Autodesk Inventor part; units mm, degrees
(part 2 of 2)
  line L199 (6.1998, 20.5703) -> (3.8425, 18.0886)
  line L200 (6.469, 17.17) -> (6.1998, 20.5703)
  spline S324 degree 2 poles (12.5142, -0.9288) (12.5142, -0.0466) (11.2141, 0.5902) knots 0 0 0 1 1 1
  spline S325 degree 2 poles (11.2141, 0.5902) (11.3534, 0.6234) (11.6187, 0.6234) knots 0 0 0 1 1 1
  spline S326 degree 2 poles (11.6187, 0.6234) (12.8393, 0.6234) (14.219, -0.8758) (14.219, -1.8774) knots 0 0 0 1 2 2 2
  spline S327 degree 2 poles (14.219, -1.8774) (14.219, -2.4347) (13.6154, -3.0516) (13.0847, -3.0516) knots 0 0 0 1 2 2 2
  spline S328 degree 2 poles (13.0847, -3.0516) (12.4147, -3.0516) (11.6386, -2.3285) knots 0 0 0 1 1 1
  spline S329 degree 2 poles (11.6386, -2.3285) (12.5142, -1.6784) (12.5142, -0.9288) knots 0 0 0 1 1 1
  spline S330 degree 2 poles (20.0897, 3.4692) (20.6005, 3.4692) (22.5176, 1.3) (23.1278, -0.2323) knots 0 0 0 1 2 2 2
  spline S331 degree 2 poles (23.1278, -0.2323) (19.7779, 2.0562) (19.7779, 3.1375) knots 0 0 0 1 1 1
  spline S332 degree 2 poles (19.7779, 3.1375) (19.7779, 3.4692) (20.0897, 3.4692) knots 0 0 0 1 1 1
  spline S333 degree 2 poles (-4.965, 3.4824) (-4.3813, 3.4824) (-2.8755, 1.8705) (-2.1126, 0.1789) knots 0 0 0 1 2 2 2
  line L201 (-2.1126, 0.1789) -> (-2.7295, 0.577)
  spline S334 degree 2 poles (-2.7295, 0.577) (-5.4692, 2.3945) (-5.4692, 3.1441) knots 0 0 0 1 1 1
  spline S335 degree 2 poles (-5.4692, 3.1441) (-5.4692, 3.4824) (-4.965, 3.4824) knots 0 0 0 1 1 1
  spline S336 degree 2 poles (-12.1956, 0.5239) (-11.5786, 0.5239) (-10.4509, -0.5839) (-10.4509, -1.4728) knots 0 0 0 1 2 2 2
  spline S337 degree 2 poles (-10.4509, -1.4728) (-12.8523, -1.0748) (-12.8523, -0.0068) knots 0 0 0 1 1 1
  spline S338 degree 2 poles (-12.8523, -0.0068) (-12.8523, 0.5239) (-12.1956, 0.5239) knots 0 0 0 1 1 1
  spline S339 degree 2 poles (-16.7793, -5.7514) (-16.7793, -5.3866) (-18.0264, -4.6303) (-19.1806, -4.3318) knots -2 -2 -2 -1 0 0 0
  spline S340 degree 2 poles (-17.3166, -6.1229) (-18.3581, -6.1229) (-19.1806, -4.3318) knots 0 0 0 1 1 1
  spline S341 degree 2 poles (-19.1806, -4.3318) (-18.0264, -4.6303) (-16.7793, -5.3866) (-16.7793, -5.7514) knots 0 0 0 1 2 2 2
  spline S342 degree 2 poles (-16.7793, -5.7514) (-16.7793, -6.1229) (-17.3166, -6.1229) knots 0 0 0 1 1 1
  spline S343 degree 2 poles (45.6088, -2.1229) (45.6088, -2.4214) (45.1112, -2.7929) (44.7265, -2.7929) knots 0 0 0 1 2 2 2
  spline S344 degree 2 poles (44.7265, -2.7929) (43.7912, -2.7929) (42.1328, -0.9156) (42.1328, -0.1196) knots 0 0 0 1 2 2 2
  spline S345 degree 2 poles (42.1328, -0.1196) (42.1328, 0.1922) (42.6038, 0.5372) (42.9952, 0.5372) knots 0 0 0 1 2 2 2
  spline S346 degree 2 poles (42.9952, 0.5372) (43.9305, 0.5372) (45.6088, -1.3401) (45.6088, -2.1229) knots 0 0 0 1 2 2 2
  spline S347 degree 2 poles (-38.0728, -0.9288) (-38.0728, -0.0466) (-39.373, 0.5902) knots 0 0 0 1 1 1
  spline S348 degree 2 poles (-39.373, 0.5902) (-39.2337, 0.6234) (-38.9684, 0.6234) knots 0 0 0 1 1 1
  spline S349 degree 2 poles (-38.9684, 0.6234) (-37.7478, 0.6234) (-36.368, -0.8758) (-36.368, -1.8774) knots 0 0 0 1 2 2 2
  spline S350 degree 2 poles (-36.368, -1.8774) (-36.368, -2.4347) (-36.9717, -3.0516) (-37.5024, -3.0516) knots 0 0 0 1 2 2 2
  spline S351 degree 2 poles (-37.5024, -3.0516) (-38.1723, -3.0516) (-38.9485, -2.3285) knots 0 0 0 1 1 1
  spline S352 degree 2 poles (-38.9485, -2.3285) (-38.0728, -1.6784) (-38.0728, -0.9288) knots 0 0 0 1 1 1
  line L202 (3.8425, 18.0886) -> (6.469, 17.17)
  spline S353 degree 2 poles (-7.28, -17.2787) (-7.0967, -17.3644) (-6.978, -17.704) (-7.1028, -18.271) (-7.3086, -18.7108) knots 0 0 0 1 2 3 3 3
  line L203 (-7.3086, -18.7108) -> (-7.5755, -19.2815)
  spline S354 degree 2 poles (-7.5755, -19.2815) (-7.867, -19.9045) (-8.3959, -20.3463) (-8.6603, -20.2226) knots 0 0 0 1 2 2 2
  spline S355 degree 2 poles (-8.6603, -20.2226) (-9.1865, -19.9764) (-8.6759, -18.8848) knots 0 0 0 1 1 1
  line L204 (-8.6759, -18.8848) -> (-8.4003, -18.2958)
  spline S356 degree 2 poles (-8.4003, -18.2958) (-8.2827, -18.0444) (-8.0517, -17.6324) (-7.9802, -17.5478) knots 0 0 0 1 2 2 2
  spline S357 degree 2 poles (-7.9802, -17.5478) (-7.6465, -17.1072) (-7.28, -17.2787) knots 0 0 0 1 1 1
  spline S358 degree 2 poles (-12.2176, -15.5395) (-11.8791, -15.1913) (-11.5755, -14.6965) (-11.5766, -14.3368) (-11.7216, -14.1958) knots -3 -3 -3 -2 -1 0 0 0
  spline S359 degree 2 poles (-11.7216, -14.1958) (-12.0118, -13.9138) (-12.4714, -14.2208) knots -1 -1 -1 0 0 0
  spline S360 degree 2 poles (-12.4714, -14.2208) (-12.5666, -14.2773) (-12.9199, -14.5909) (-13.1132, -14.7899) knots -2 -2 -2 -1 0 0 0
  line L205 (-13.1132, -14.7899) -> (-13.5665, -15.2562)
  spline S361 degree 2 poles (-13.5665, -15.2562) (-14.4064, -16.1205) (-13.9898, -16.5254) knots -1 -1 -1 0 0 0
  spline S362 degree 2 poles (-13.9898, -16.5254) (-13.7805, -16.7288) (-13.1361, -16.4846) (-12.6567, -15.9913) knots -2 -2 -2 -1 0 0 0
  line L206 (-12.6567, -15.9913) -> (-12.2176, -15.5395)
  spline S363 degree 2 poles (-11.7843, -16.3959) (-12.1308, -16.7523) (-13.001, -17.0713) (-13.839, -16.9259) (-14.1375, -16.6358) knots -3 -3 -3 -2 -1 0 0 0
  spline S364 degree 2 poles (-14.1375, -16.6358) (-14.3655, -16.4142) (-14.4588, -16.0334) knots -1 -1 -1 0 0 0
  spline S365 degree 2 poles (-14.4588, -16.0334) (-14.5129, -15.8236) (-14.497, -15.3594) (-14.3622, -14.9222) (-14.1024, -14.5056) (-13.9211, -14.3191) knots -4 -4 -4 -3 -2 -1 0 0 0
  spline S366 degree 2 poles (-13.9211, -14.3191) (-13.625, -14.0144) (-12.9266, -13.6897) (-12.6095, -13.7077) knots -2 -2 -2 -1 0 0 0
  spline S367 degree 2 poles (-12.6095, -13.7077) (-12.387, -13.6861) (-12.0199, -13.7728) (-11.7068, -13.9442) (-11.5908, -14.057) knots -3 -3 -3 -2 -1 0 0 0
  spline S368 degree 2 poles (-11.5908, -14.057) (-11.2923, -14.347) (-11.1417, -15.1665) (-11.4419, -16.0435) (-11.7843, -16.3959) knots -3 -3 -3 -2 -1 0 0 0
  spline S369 degree 2 poles (-31.5521, 3.5488) (-30.4576, 3.5488) (-28.8788, 0.4642) knots 0 0 0 1 1 1
  spline S370 degree 2 poles (-28.8788, 0.4642) (-30.3912, 1.3398) (-31.9567, 2.8191) (-31.9567, 3.1972) knots 0 0 0 1 2 2 2
  spline S371 degree 2 poles (-31.9567, 3.1972) (-31.9567, 3.3498) (-31.7246, 3.5488) (-31.5521, 3.5488) knots 0 0 0 1 2 2 2
  point P0 (0, 0)
  constraints: 1 other
extrude "Extrusion2" add sketch "Skizze1" against normal blind 2 contours L187 L188 A0 L189 L190 L191 A1 L192 | L200 L202 L199 | S324 S325 S326 S327 S328 S329 | S330 S331 S332 | S333 L201 S334 S335 | S336 S337 S338 | S342 S340 S339 | S343 S344 S345 S346 | S347 S348 S349 S350 S351 S352 | S353 L203 S354 S355 L204 S356 S357 | L206 S362 S361 L205 S360 S359 S358 | S369 S370 S371
sketch "Skizze2" plane through (0, 0, -2) normal (0, 0, -1) x (-1, 0, 0)
  arc A0 (26.5702, 11) -> (-26.5702, 11) centre (0, 0) ccw construction
  line L0 (-26.5702, 11) -> (-52, 11) construction
  line L1 (-52, 11) -> (-52, -11) construction
  line L2 (-52, -11) -> (-26.5702, -11) construction
  arc A1 (-26.5702, -11) -> (26.5702, -11) centre (0, 0) ccw construction
  line L3 (26.5702, -11) -> (52, -11) construction
  line L4 (52, -11) -> (52, 11) construction
  line L5 (52, 11) -> (26.5702, 11) construction
  arc A2 (27.8748, 13) -> (-27.8748, 13) centre (0, 0) ccw
  line L6 (27.8748, 13) -> (54, 13)
  line L7 (54, 13) -> (54, -13)
  line L8 (54, -13) -> (27.8748, -13)
  arc A3 (-27.8748, -13) -> (27.8748, -13) centre (0, 0) ccw
  line L9 (-27.8748, -13) -> (-54, -13)
  line L10 (-54, -13) -> (-54, 13)
  line L11 (-54, 13) -> (-27.8748, 13)
  arc A4 (26.77, 11.3) -> (-26.77, 11.3) centre (0, 0) ccw
  line L12 (26.77, 11.3) -> (52.3, 11.3)
  line L13 (52.3, 11.3) -> (52.3, -11.3)
  line L14 (52.3, -11.3) -> (26.77, -11.3)
  arc A5 (-26.77, -11.3) -> (26.77, -11.3) centre (0, 0) ccw
  line L15 (-26.77, -11.3) -> (-52.3, -11.3)
  line L16 (-52.3, -11.3) -> (-52.3, 11.3)
  line L17 (-52.3, 11.3) -> (-26.77, 11.3)
  point P0 (0, 0)
  dimension "d4" = 2
  dimension "d7" = 0.3
  constraints: 24 end point, 8 point on circle, 4 centre point, 14 other
  measures "d4" radial gap between concentric circles of A0 A2
  measures "d7" radial gap between concentric circles of A0 A4
extrude "Extrusion4" add sketch "Skizze2" against normal blind 4
sketch "Skizze3" plane through (0, 0, -2) normal (0, 0, -1) x (-1, 0, 0)
  line L0 (-52.3, -11.3) -> (-52.3, 11.3) construction
  line L1 (-52.3, 11.3) -> (-26.77, 11.3) construction
  line L2 (-50, 9) -> (-50, -9) construction
  line L3 (-25.1982, 9) -> (-50, 9) construction
  line L4 (19.4526, -3.7813) -> (20.0231, -2.6005) construction
  line L5 (15.3597, -1.8575) -> (15.3597, -1.9596) construction
  line L6 (15.9169, -0.7033) -> (16.8191, 0.6964) construction
  line L7 (16.8191, 0.6964) -> (19.5388, 0.975) construction
  line L8 (19.5388, 0.975) -> (18.3713, -0.6635) construction
  line L9 (20.7196, -1.035) -> (21.7876, 0.6964) construction
  line L10 (21.7876, 0.6964) -> (24.3415, 0.975) construction
  line L11 (24.3415, 0.975) -> (21.907, -3.3302) construction
  line L12 (25.4227, -1.8575) -> (25.4227, -2.4944) construction
  line L13 (-2.0797, -0.3915) -> (-3.161, -0.6967) construction
  line L14 (-1.0184, -1.8575) -> (-1.0184, -2.262) construction
  line L15 (5.5886, -2.0499) -> (5.5355, -2.5474) construction
  line L16 (8.2553, -1.8443) -> (8.2553, -2.4811) construction
  line L17 (1.2105, -3.6088) -> (-0.9189, -3.8211) construction
  line L18 (-41.4628, 0.3514) -> (-39.5457, 0.975) construction
  line L19 (-39.5457, 0.975) -> (-39.0217, 0.975) construction
  line L20 (-39.0217, 0.975) -> (-39.8443, -0.637) construction
  line L21 (-37.8675, -1.8575) -> (-37.8675, -2.4944) construction
  line L22 (8.4237, -11.8985) -> (-8.4237, -11.8985) construction
  line L23 (-8.4237, -11.8985) -> (-8.4237, -10.2137) construction
  line L24 (-8.4237, -10.2137) -> (8.4237, -10.2137) construction
  line L25 (8.4237, -10.2137) -> (8.4237, -11.8985) construction
  line L26 (8.4237, 8.1078) -> (-8.4237, 8.1078) construction
  line L27 (-8.4237, 8.1078) -> (-8.4237, 9.7925) construction
  line L28 (-8.4237, 9.7925) -> (8.4237, 9.7925) construction
  line L29 (8.4237, 9.7925) -> (8.4237, 8.1078) construction
  line L30 (-36.501, 0.6698) -> (-34.1195, 0.9617) construction
  line L31 (-34.1195, 0.9617) -> (-34.0068, 0.9617) construction
  line L32 (-34.0068, 0.9617) -> (-34.9421, -0.763) construction
  line L33 (-33.1444, -1.8575) -> (-33.1444, -1.9262) construction
  line L34 (-27.8708, 0.9418) -> (-27.0151, 0.9617) construction
  line L35 (-27.0151, 0.9617) -> (-27.8907, -0.4512) construction
  line L36 (-26.0399, -1.8575) -> (-26.0399, -2.4944) construction
  line L37 (-33.0449, -2.4944) -> (-33.1444, -2.4944) construction
  line L38 (-50, 9) -> (-50, -9) construction
  line L39 (-50, -9) -> (-25.1982, -9) construction
  arc A0 (-25.1982, -9) -> (25.1982, -9) centre (0, 0) ccw construction
  line L40 (25.1982, -9) -> (50, -9) construction
  line L41 (50, -9) -> (50, 9) construction
  line L42 (50, 9) -> (25.1982, 9) construction
  arc A1 (25.1982, 9) -> (-25.1982, 9) centre (0, 0) ccw construction
  line L43 (-25.1982, 9) -> (-50, 9) construction
  line L44 (10.3827, -18.585) -> (11.6479, -17.7113) construction
  line L45 (11.8599, -16.9959) -> (11.7864, -16.8184) construction
  line L46 (11.7864, -16.8184) -> (11.9387, -16.7133) construction
  line L47 (11.9387, -16.7133) -> (12.5299, -18.012) construction
  line L48 (12.5299, -18.012) -> (10.3324, -19.5294) construction
  line L49 (4.5777, -20.9876) -> (6.0592, -20.5763) construction
  line L50 (6.4937, -19.9698) -> (6.4825, -19.778) construction
  line L51 (6.4825, -19.778) -> (6.6607, -19.7285) construction
  line L52 (6.6607, -19.7285) -> (6.7941, -21.1492) construction
  line L53 (6.7941, -21.1492) -> (4.2209, -21.8635) construction
  line L54 (-11.3462, -15.6476) -> (-11.4647, -15.521) construction
  line L55 (-12.2821, -14.5759) -> (-12.2616, -14.6359) construction
  line L56 (-12.2616, -14.6359) -> (-12.1277, -14.855) construction
  line L57 (-15.0012, -14.9954) -> (-15.1236, -14.8645) construction
  line L58 (-15.1236, -14.8645) -> (-13.9041, -13.7229) construction
  line L59 (-13.9041, -13.7229) -> (-13.7796, -13.8558) construction
  line L60 (-12.876, -15.2229) -> (-12.9953, -14.9982) construction
  line L61 (-10.5425, -14.6538) -> (-10.422, -14.7825) construction
  line L62 (-10.422, -14.7825) -> (-11.3462, -15.6476) construction
  line L63 (-10.2693, -15.0123) -> (-10.3867, -14.9232) construction
  line L64 (-10.3867, -14.9232) -> (-10.2714, -14.7712) construction
  line L65 (-10.2714, -14.7712) -> (-8.4825, -16.1288) construction
  line L66 (-8.4825, -16.1288) -> (-8.5299, -16.1912) construction
  line L67 (-8.5299, -16.1912) -> (-7.5089, -16.6901) construction
  line L68 (-7.5089, -16.6901) -> (-6.5286, -19.8907) construction
  line L69 (-6.5286, -19.8907) -> (-5.908, -18.621) construction
  line L70 (-6.2567, -17.5112) -> (-6.1742, -17.3424) construction
  line L71 (-6.1742, -17.3424) -> (-4.5695, -18.1267) construction
  line L72 (-4.5695, -18.1267) -> (-4.6533, -18.2981) construction
  line L73 (-4.6533, -18.2981) -> (-4.7312, -18.26) construction
  line L74 (-5.7377, -18.7267) -> (-6.8279, -20.9572) construction
  line L75 (-6.8279, -20.9572) -> (-6.9681, -20.8887) construction
  line L76 (-6.9681, -20.8887) -> (-8.2125, -16.9253) construction
  line L77 (-8.2125, -16.9253) -> (-9.0755, -18.691) construction
  line L78 (-8.6257, -19.8309) -> (-8.7082, -19.9996) construction
  line L79 (-8.7082, -19.9996) -> (-10.3934, -19.176) construction
  line L80 (-10.3934, -19.176) -> (-10.3109, -19.0072) construction
  line L81 (-9.3091, -18.728) -> (-8.4652, -17.0013) construction
  line L82 (-8.8001, -16.2714) -> (-8.8858, -16.2295) construction
  line L83 (-8.8858, -16.2295) -> (-8.83, -16.1154) construction
  line L84 (-9.5066, -16.3022) -> (-10.7017, -17.8769) construction
  line L85 (-10.5969, -18.6712) -> (-10.4795, -18.7603) construction
  line L86 (-10.4795, -18.7603) -> (-10.5983, -18.9169) construction
  line L87 (-10.5983, -18.9169) -> (-12.3872, -17.5593) construction
  line L88 (-12.3872, -17.5593) -> (-12.2684, -17.4028) construction
  line L89 (-12.2684, -17.4028) -> (-12.151, -17.4919) construction
  line L90 (-1.5804, -18.6594) -> (-1.4224, -18.6945) construction
  line L91 (-1.4224, -18.6945) -> (-1.423, -18.698) construction
  line L92 (-1.423, -18.698) -> (2.097, -18.7064) construction
  line L93 (2.097, -18.7064) -> (2.0937, -20.1226) construction
  line L94 (2.0937, -20.1226) -> (1.9289, -20.1222) construction
  line L95 (0.5272, -18.8934) -> (-0.0913, -18.892) construction
  line L96 (-0.0913, -18.892) -> (-0.0949, -20.4064) construction
  line L97 (-0.0949, -20.4064) -> (0.0323, -20.4067) construction
  line L98 (0.8586, -19.3306) -> (1.0435, -19.3311) construction
  line L99 (1.0435, -19.3311) -> (1.038, -21.6605) construction
  line L100 (1.038, -21.6605) -> (0.8559, -21.6601) construction
  line L101 (-0.0057, -20.5916) -> (-0.0953, -20.5914) construction
  line L102 (-0.0953, -20.5914) -> (-0.0987, -22.0104) construction
  line L103 (-0.0987, -22.0104) -> (0.41, -22.0116) construction
  line L104 (1.9998, -20.7062) -> (2.1819, -20.7066) construction
  line L105 (2.1819, -20.7066) -> (2.1783, -22.2066) construction
  line L106 (2.1783, -22.2066) -> (-1.6222, -22.1976) construction
  line L107 (-1.6222, -22.1976) -> (-1.6304, -22.0068) construction
  line L108 (-1.6304, -22.0068) -> (-1.4859, -22.0072) construction
  line L109 (-0.9181, -21.4334) -> (-0.9134, -19.4565) construction
  line L110 (-1.4571, -18.8889) -> (-1.7278, -20.403) construction
  line L111 (-1.7278, -20.403) -> (-1.8971, -20.3654) construction
  line L112 (-1.9582, -20.8403) -> (-1.7889, -20.8779) construction
  line L113 (-0.0057, 17.1193) -> (0.1705, 17.1809) construction
  line L114 (0.1705, 17.1809) -> (0.236, 16.9937) construction
  line L115 (0.236, 16.9937) -> (-3.6019, 15.6514) construction
  line L116 (-3.6019, 15.6514) -> (-3.6674, 15.8386) construction
  line L117 (-3.6674, 15.8386) -> (-3.1663, 16.0139) construction
  line L118 (-3.4924, 17.7414) -> (-3.6873, 17.9452) construction
  line L119 (-3.6873, 17.9452) -> (-6.4844, 16.9668) construction
  line L120 (-6.4844, 16.9668) -> (-6.5278, 16.4017) construction
  line L121 (-5.1871, 15.3071) -> (-5.1216, 15.1199) construction
  line L122 (-5.1216, 15.1199) -> (-7.8142, 14.1781) construction
  line L123 (-7.8142, 14.1781) -> (-7.8796, 14.3653) construction
  line L124 (-6.6813, 16.8053) -> (-6.2399, 22.2929) construction
  line L125 (-6.2399, 22.2929) -> (-6.0637, 22.3545) construction
  line L126 (-6.0637, 22.3545) -> (-1.3895, 17.5067) construction
  line L127 (18.2568, 9.2337) -> (18.1666, 9.3837) construction
  line L128 (16.7022, 11.6138) -> (16.7786, 11.3738) construction
  line L129 (16.7786, 11.3738) -> (16.8901, 10.9848) construction
  line L130 (11.1824, 12.0981) -> (11.0921, 12.248) construction
  line L131 (11.0921, 12.248) -> (13.8712, 13.9202) construction
  line L132 (13.8712, 13.9202) -> (13.9614, 13.7702) construction
  line L133 (15.4289, 10.6298) -> (15.2852, 11.1288) construction
  line L134 (20.2209, 10.6198) -> (20.3111, 10.4698) construction
  line L135 (20.3111, 10.4698) -> (18.2568, 9.2337) construction
  line L136 (-11.0519, 15.7859) -> (-11.133, 15.6504) construction
  line L137 (-15.5268, 15.2762) -> (-15.7383, 14.9757) construction
  line L138 (-15.7383, 14.9757) -> (-11.3688, 11.9001) construction
  line L139 (-9.6004, 12.2033) -> (-8.9893, 13.0714) construction
  line L140 (-8.9893, 13.0714) -> (-8.8271, 12.9573) construction
  line L141 (-8.8271, 12.9573) -> (-12.3459, 7.9582) construction
  line L142 (-12.3459, 7.9582) -> (-12.508, 8.0723) construction
  line L143 (-12.508, 8.0723) -> (-11.9037, 8.931) construction
  line L144 (-12.2116, 10.7028) -> (-16.581, 13.7784) construction
  line L145 (-16.581, 13.7784) -> (-16.8396, 13.4111) construction
  line L146 (-15.672, 9.2222) -> (-15.7727, 9.0791) construction
  line L147 (-15.7727, 9.0791) -> (-18.6778, 11.1239) construction
  line L148 (-18.6778, 11.1239) -> (-13.9569, 17.8307) construction
  line L149 (-13.9569, 17.8307) -> (-11.0519, 15.7859) construction
  line L150 (42.9418, -0.8758) -> (43.3531, -0.04) construction
  line L151 (43.3531, -0.04) -> (42.6234, -0.0599) construction
  line L152 (42.6234, -0.0599) -> (42.9219, 0.8025) construction
  line L153 (42.9219, 0.8025) -> (43.8174, 0.8224) construction
  line L154 (43.8174, 0.8224) -> (44.6931, 2.5405) construction
  line L155 (44.6931, 2.5405) -> (47.2138, 2.8456) construction
  line L156 (47.2138, 2.8456) -> (46.2387, 0.9285) construction
  line L157 (46.2387, 0.9285) -> (47.5455, 0.975) construction
  line L158 (47.5455, 0.975) -> (47.2403, 0.1259) construction
  line L159 (47.2403, 0.1259) -> (45.8009, 0.0595) construction
  line L160 (45.8009, 0.0595) -> (45.1707, -1.1743) construction
  line L161 (47.9501, -1.8575) -> (47.9501, -2.4944) construction
  line L162 (42.4642, -2.3882) -> (42.4642, -2.4944) construction
  line L163 (33.9534, -2.0831) -> (33.9534, -2.4944) construction
  line L164 (29.635, 0.3249) -> (28.4078, -0.3982) construction
  line L165 (33.9534, -1.8575) -> (33.9534, -2.0831) construction
  line L166 (42.4642, -1.8575) -> (42.4642, -2.3882) construction
  line L167 (6.4558, 16.974) -> (10.8024, 21.0536) construction
  line L168 (10.8024, 21.0536) -> (13.3825, 20.076) construction
  line L169 (13.3825, 20.076) -> (13.3164, 19.9014) construction
  line L170 (13.3164, 19.9014) -> (13.0764, 19.9924) construction
  line L171 (11.4367, 19.2538) -> (9.994, 15.4462) construction
  line L172 (10.7326, 13.8065) -> (10.9726, 13.7156) construction
  line L173 (10.9726, 13.7156) -> (10.9024, 13.5301) construction
  line L174 (10.9024, 13.5301) -> (6.6693, 15.134) construction
  line L175 (6.6693, 15.134) -> (6.7396, 15.3194) construction
  line L176 (6.7396, 15.3194) -> (7.0233, 15.212) construction
  line L177 (8.6576, 15.9526) -> (10.3441, 20.4038) construction
  line L178 (10.3441, 20.4038) -> (10.3277, 20.41) construction
  line L179 (10.3277, 20.41) -> (5.3056, 15.6507) construction
  line L180 (5.3056, 15.6507) -> (5.1474, 15.7106) construction
  line L181 (5.1474, 15.7106) -> (4.4991, 22.5935) construction
  line L182 (4.4991, 22.5935) -> (4.4827, 22.5997) construction
  line L183 (4.4827, 22.5997) -> (2.885, 18.3831) construction
  line L184 (3.8158, 16.4272) -> (3.7455, 16.2418) construction
  line L185 (3.7455, 16.2418) -> (0.6744, 17.4054) construction
  line L186 (0.6744, 17.4054) -> (0.7447, 17.5909) construction
  line L187 (0.7447, 17.5909) -> (0.8101, 17.5661) construction
  line L188 (2.6838, 18.4281) -> (4.0562, 22.0502) construction
  line L189 (3.3176, 23.6899) -> (3.0885, 23.7767) construction
  line L190 (3.0885, 23.7767) -> (3.1546, 23.9513) construction
  line L191 (3.1546, 23.9513) -> (5.8875, 22.9158) construction
  line L192 (5.8875, 22.9158) -> (6.4558, 16.974) construction
  line L193 (-8.1229, -1.8575) -> (-8.1229, -2.4944) construction
  line L194 (-16.6336, -2.0831) -> (-16.6336, -2.4944) construction
  line L195 (-23.7182, -3.5623) -> (-25.8078, -3.8476) construction
  line L196 (-16.6336, -1.8575) -> (-16.6336, -2.0831) construction
  line L197 (-52.3, 11.3) -> (-26.77, 11.3) construction
  arc A2 (26.77, 11.3) -> (-26.77, 11.3) centre (0, 0) ccw construction
  line L198 (26.77, 11.3) -> (52.3, 11.3) construction
  line L199 (52.3, 11.3) -> (52.3, -11.3) construction
  line L200 (52.3, -11.3) -> (26.77, -11.3) construction
  arc A3 (-26.77, -11.3) -> (26.77, -11.3) centre (0, 0) ccw construction
  line L201 (-26.77, -11.3) -> (-52.3, -11.3) construction
  line L202 (-52.3, -11.3) -> (-52.3, 11.3) construction
  arc A4 (27.8748, 13) -> (-27.8748, 13) centre (0, 0) ccw construction
  line L203 (-54, 13) -> (-27.8748, 13) construction
  line L204 (-54, -13) -> (-54, 13) construction
  line L205 (-27.8748, -13) -> (-54, -13) construction
  arc A5 (-27.8748, -13) -> (27.8748, -13) centre (0, 0) ccw construction
  line L206 (54, -13) -> (27.8748, -13) construction
  line L207 (54, 13) -> (54, -13) construction
  line L208 (27.8748, 13) -> (54, 13) construction
  line L209 (-26.77, 11.3) -> (-52.3, 11.3) construction
  line L210 (-41.4628, 12.3911) -> (-40.9374, 12.3911)
  line L211 (-40.9374, 12.3911) -> (-40.9374, 7.5497)
  line L212 (-40.9374, 7.5497) -> (-41.4628, 7.5497)
  line L213 (-41.4628, 7.5497) -> (-41.4628, 12.3911)
  line L214 (-41.4628, -7.8889) -> (-40.9374, -7.8889)
  line L215 (-40.9374, -7.8889) -> (-40.9374, -12.6122)
  line L216 (-40.9374, -12.6122) -> (-41.4628, -12.6122)
  line L217 (-41.4628, -12.6122) -> (-41.4628, -7.8889)
  line L218 (39.535, 12.2033) -> (40.1282, 12.2033)
  line L219 (40.1282, 12.2033) -> (40.1282, 8.0723)
  line L220 (40.1282, 8.0723) -> (39.535, 8.0723)
  line L221 (39.535, 8.0723) -> (39.535, 12.2033)
  line L222 (39.535, -7.8889) -> (40.1282, -7.8889)
  line L223 (40.1282, -7.8889) -> (40.1282, -11.896)
  line L224 (40.1282, -11.896) -> (39.535, -11.896)
  line L225 (39.535, -11.896) -> (39.535, -7.8889)
  line L226 (-4.7561, 16.8236) -> (-5.1557, 16.8236)
  line L227 (-5.1557, 16.8236) -> (-5.1557, 18.0886)
  line L228 (-5.1557, 18.0886) -> (-4.7561, 18.0886)
  line L229 (-4.7561, 18.0886) -> (-4.7561, 16.8236)
  line L230 (37.8919, 1.6091) -> (38.2709, 1.6091)
  line L231 (38.2709, 1.6091) -> (38.2709, 0.2784)
  line L232 (38.2709, 0.2784) -> (37.8919, 0.2784)
  line L233 (37.8919, 0.2784) -> (37.8919, 1.6091)
  line L234 (5.8875, 1.6091) -> (3.7455, 1.6091)
  line L235 (3.7455, 1.6091) -> (3.7455, 1.8871)
  line L236 (3.7455, 1.8871) -> (5.8875, 1.8871)
  line L237 (5.8875, 1.8871) -> (5.8875, 1.6091)
  line L238 (-12.5044, 1.2992) -> (-12.2116, 1.2992)
  line L239 (-12.2116, 1.2992) -> (-12.2116, 0.2784)
  line L240 (-12.2116, 0.2784) -> (-12.5044, 0.2784)
  line L241 (-12.5044, 0.2784) -> (-12.5044, 1.2992)
  line L242 (-43.6384, 1.2992) -> (-43.4506, 1.2992)
  line L243 (-43.4506, 1.2992) -> (-43.4506, -0.2951)
  line L244 (-43.4506, -0.2951) -> (-43.6384, -0.2951)
  line L245 (-43.6384, -0.2951) -> (-43.6384, 1.2992)
  line L246 (-19.3718, 1.8871) -> (-21.2265, 1.8871)
  line L247 (-21.2265, 1.8871) -> (-21.2265, 1.6091)
  line L248 (-21.2265, 1.6091) -> (-19.3718, 1.6091)
  line L249 (-19.3718, 1.6091) -> (-19.3718, 1.8871)
  line L250 (11.4367, 1.6091) -> (11.8018, 1.6091)
  line L251 (11.8018, 1.6091) -> (11.8018, -0.2951)
  line L252 (11.8018, -0.2951) -> (11.4367, -0.2951)
  line L253 (11.4367, -0.2951) -> (11.4367, 1.6091)
  line L254 (32.7025, 1.8871) -> (29.8937, 1.8871)
  line L255 (29.8937, 1.8871) -> (29.8937, 1.6091)
  line L256 (29.8937, 1.6091) -> (32.7025, 1.6091)
  line L257 (32.7025, 1.6091) -> (32.7025, 1.8871)
  line L258 (8.6576, -21.5522) -> (8.2951, -21.5522)
  line L259 (8.2951, -21.5522) -> (8.2951, -19.3861)
  line L260 (8.2951, -19.3861) -> (8.6576, -19.3861)
  line L261 (8.6576, -19.3861) -> (8.6576, -21.5522)
  line L262 (13.8712, -17.8769) -> (13.6679, -17.8769)
  line L263 (13.6679, -17.8769) -> (13.6679, -15.7541)
  line L264 (13.6679, -15.7541) -> (13.8712, -15.7541)
  line L265 (13.8712, -15.7541) -> (13.8712, -17.8769)
  point P0 (0, 0)
  point P1 (17.3896, -6.5408)
  point P2 (16.0695, -5.7514)
  point P3 (16.912, -3.7614)
  point P4 (15.3006, -2.5283)
  point P5 (11.1342, -3.8343)
  point P6 (8.2951, -2.0963)
  point P7 (12.7262, 0.9617)
  point P8 (14.6499, 0.0065)
  point P9 (10.5239, -1.8443)
  point P10 (12.4808, -2.9189)
  point P11 (17.5687, -2.4413)
  point P12 (18.1392, -2.9388)
  point P13 (21.6151, -3.8741)
  point P14 (-8.103, -2.1892)
  point P15 (-3.4927, 0.975)
  point P16 (-1.6088, -0.0068)
  point P17 (-3.4529, -0.7497)
  point P18 (-3.5855, -0.637)
  point P19 (-3.4728, -0.0466)
  point P20 (-4.1096, 0.4907)
  point P21 (-5.9272, -1.4595)
  point P22 (-3.9703, -2.899)
  point P23 (2.2055, 3.4559)
  point P24 (5.6019, 4.1325)
  point P25 (6.2586, 3.31)
  point P26 (3.9899, 0.8357)
  point P27 (5.3166, 0.975)
  point P28 (7.2934, 0.0463)
  point P29 (4.4941, -1.2937)
  point P30 (6.0662, -2.8857)
  point P31 (4.7262, -3.8476)
  point P32 (3.1342, -2.8857)
  point P33 (3.3597, -1.8708)
  point P34 (2.3846, -1.3866)
  point P35 (3.0281, -1.0483)
  point P36 (5.0712, -0.239)
  point P37 (4.0894, 0.2784)
  point P38 (3.6383, 0.2453)
  point P39 (3.2072, 0.1458)
  point P40 (2.7561, -0.0333)
  point P41 (2.2785, -0.3186)
  point P42 (1.7478, -0.6967)
  point P43 (1.3697, -1.7846)
  point P44 (1.2171, -2.7133)
  point P45 (-1.0383, -2.7929)
  point P46 (-1.0324, -2.5024)
  point P47 (-5.3036, -3.8343)
  point P48 (-42.6502, -2.2953)
  point P49 (-46.0134, -3.8343)
  point P50 (-47.9902, -2.2622)
  point P51 (-43.1013, 0.9882)
  point P52 (-40.4877, -2.3086)
  point P53 (-39.9106, -2.7796)
  point P54 (-41.2506, -3.8343)
  point P55 (-37.8476, -2.5806)
  point P56 (-35.5258, -2.2887)
  point P57 (-35.0482, -2.6934)
  point P58 (-31.9371, -1.035)
  point P59 (-32.7398, -0.4114)
  point P60 (-30.8957, 0.975)
  point P61 (-30.166, 0.5372)
  point P62 (-30.5839, -0.4579)
  point P63 (-28.753, -2.2356)
  point P64 (-28.0764, -2.7398)
  point P65 (-29.6685, -3.8476)
  point P66 (-31.0283, -2.8592)
  point P67 (-29.6154, -0.7763)
  point P68 (-31.1278, -1.0682)
  point P69 (-36.4214, -3.8476)
  point P70 (-36.3683, 2.0761)
  point P71 (-35.5258, 3.164)
  point P72 (-34.3318, 2.8987)
  point P73 (-33.3302, 3.111)
  point P74 (-34.9885, 1.7909)
  point P75 (10.2153, -18.8411)
  point P76 (10.5063, -17.8078)
  point P77 (10.6659, -17.3217)
  point P78 (10.6898, -17.2139)
  point P79 (10.5135, -16.3381)
  point P80 (9.4182, -16.0795)
  point P81 (9.0613, -17.348)
  point P82 (9.2392, -17.4886)
  point P83 (9.2242, -17.4567)
  point P84 (9.1838, -17.3371)
  point P85 (9.3851, -16.8047)
  point P86 (10.0476, -16.9198)
  point P87 (9.8798, -17.6889)
  point P88 (8.9087, -17.4779)
  point P89 (8.7696, -16.717)
  point P90 (9.468, -15.7956)
  point P91 (11.2719, -15.8495)
  point P92 (11.422, -16.494)
  point P93 (11.3538, -16.787)
  point P94 (10.973, -17.4714)
  point P95 (10.4994, -18.3675)
  point P96 (4.3357, -21.1747)
  point P97 (4.9489, -20.2936)
  point P98 (5.2589, -19.8867)
  point P99 (5.3168, -19.7926)
  point P100 (5.437, -18.9074)
  point P101 (4.4867, -18.3043)
  point P102 (3.7342, -19.3861)
  point P103 (3.8562, -19.5771)
  point P104 (3.8525, -19.5422)
  point P105 (3.8534, -19.4159)
  point P106 (4.218, -18.9788)
  point P107 (4.8063, -19.3044)
  point P108 (4.3959, -19.9762)
  point P109 (3.5474, -19.4589)
  point P110 (3.6651, -18.6944)
  point P111 (4.6268, -18.0525)
  point P112 (6.3136, -18.694)
  point P113 (6.2443, -19.3522)
  point P114 (6.084, -19.6066)
  point P115 (5.5, -20.1287)
  point P116 (4.7592, -20.8202)
  point P117 (-11.2118, -14.7973)
  point P118 (-11.722, -13.4657)
  point P119 (-12.2788, -13.1754)
  point P120 (-12.6198, -13.2848)
  point P121 (-12.7314, -13.5674)
  point P122 (-12.3399, -14.4677)
  point P123 (-11.7262, -16.0113)
  point P124 (-12.002, -16.6218)
  point P125 (-12.7404, -16.8775)
  point P126 (-13.7413, -16.3497)
  point P127 (-14.2288, -15.5075)
  point P128 (-14.4675, -15.058)
  point P129 (-14.1201, -14.6298)
  point P130 (-13.5983, -16.2317)
  point P131 (-12.6478, -16.4267)
  point P132 (-12.5235, -16.1281)
  point P133 (-13.3477, -14.275)
  point P134 (-13.4982, -13.5052)
  point P135 (-13.2667, -13.0589)
  point P136 (-11.583, -13.3435)
  point P137 (-11.0187, -14.3988)
  point P138 (-10.9072, -14.6745)
  point P139 (7.2018, -17.1047)
  point P140 (8.2787, -17.1082)
  point P141 (9.3178, -18.1154)
  point P142 (9.2645, -19.9112)
  point P143 (8.7637, -20.3753)
  point P144 (6.6188, -19.378)
  point P145 (11.5908, -14.057)
  point P146 (12.6095, -13.7077)
  point P147 (13.9211, -14.3191)
  point P148 (14.4588, -16.0334)
  point P149 (14.1375, -16.6358)
  point P150 (11.7843, -16.3959)
  point P151 (-11.352, -17.3761)
  point P152 (-10.844, -16.7784)
  point P153 (-10.1284, -15.7541)
  point P154 (-10.0181, -15.3553)
  point P155 (-5.8961, -17.8001)
  point P156 (-9.1266, -19.467)
  point P157 (-8.9103, -19.6628)
  point P158 (-2.2628, -21.5188)
  point P159 (-3.7414, -21.8447)
  point P160 (-5.3, -19.6244)
  point P161 (-4.1318, -18.4036)
  point P162 (-3.0964, -18.2605)
  point P163 (-2.2321, -18.7811)
  point P164 (-2.0531, -18.9215)
  point P165 (1.5841, -19.2803)
  point P166 (1.2581, -19.0194)
  point P167 (0.6284, -20.0844)
  point P168 (0.7999, -19.6831)
  point P169 (0.5718, -20.8386)
  point P170 (1.4744, -21.6876)
  point P171 (1.831, -21.2029)
  point P172 (-1.9611, -19.7739)
  point P173 (-3.0958, -18.4442)
  point P174 (-4.3602, -19.8717)
  point P175 (-4.3171, -21.2638)
  point P176 (-3.6437, -21.671)
  point P177 (-2.4531, -21.4291)
  point P178 (-2.5894, 16.6791)
  point P179 (-3.3108, 17.5577)
  point P180 (-6.4552, 15.8585)
  point P181 (-5.7583, 15.2618)
  point P182 (-7.1511, 15.0033)
  point P183 (18.9593, 10.6912)
  point P184 (18.4944, 13.6929)
  point P185 (17.4368, 14.5679)
  point P186 (16.6166, 14.4828)
  point P187 (16.2351, 13.9401)
  point P188 (16.6309, 11.8568)
  point P189 (17.2142, 8.5792)
  point P190 (16.4253, 7.4917)
  point P191 (14.9509, 7.3058)
  point P192 (13.1864, 8.7562)
  point P193 (12.5687, 10.6652)
  point P194 (12.2833, 11.6713)
  point P195 (12.9828, 12.3644)
  point P196 (13.3483, 8.8264)
  point P197 (15.3222, 7.9786)
  point P198 (15.7526, 8.5984)
  point P199 (14.869, 12.771)
  constraints: 112 end point, 28 parallel, 14 horizontal, 14 perpendicular, 10 point on line, 324 other
ref_plane "Arbeitsebene1" through (-52, -28.7572, -1) normal (0, 0, -1) x (0, 1, 0)
extrude "Extrusion5" add sketch "Skizze3" against normal blind 1
